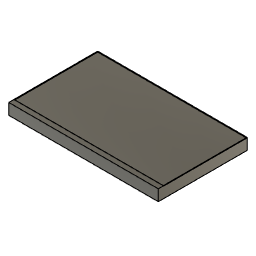
Final product (Autodesk Fusion 360 archive; units mm, degrees)
design "Écran 1"
Autodesk Fusion 360 part; units mm, degrees
sketch "Esquisse1" plane through (0, 0, 0) normal (0, 0, 1) x (1, 0, 0)
  line L0 (269, 160) -> (-269, 160)
  line L1 (-269, 160) -> (-269, -160)
  line L2 (-269, -160) -> (269, -160)
  line L3 (269, -160) -> (269, 160)
  line L4 (269, 160) -> (-269, -160) construction
  line L5 (-269, 160) -> (269, -160) construction
  dimension "d1" = 538
  dimension "d2" = 320
  constraint horizontal L0
  constraint perpendicular L0 L1
  constraint parallel L0 L2
  constraint parallel L1 L3
  constraint coincident L4 origin
  constraint coincident L5 origin
  measures "d1" distance of L1.end L2.end
  measures "d2" distance of L0.end L1.end
extrude "Extrusion1" add sketch "Esquisse1" along normal blind 40 makes body 1
sketch "Esquisse2" plane through (0, 0, 40) normal (0, 0, 1) x (-1, 0, 0)
  line L0 (-269, 160) -> (-269, -160)
  line L1 (-269, -160) -> (269, -160)
  line L2 (269, -160) -> (269, 160)
  line L3 (269, 160) -> (-269, 160)
  line L4 (268, -159) -> (-268, -159)
  line L5 (-268, -159) -> (-268, 141)
  line L6 (-268, 141) -> (268, 141)
  line L7 (268, 141) -> (268, -159)
  dimension "d5" = 536
  dimension "d6" = 300
  dimension "d7" = 1
  dimension "d8" = 1
  constraint horizontal L4
  constraint vertical L5
  constraint horizontal L6
  constraint vertical L7
  measures "d5" distance of L4.start L4.end
  measures "d6" distance of L4.start L6.end
  measures "d7" distance of L1 L4
  measures "d8" distance of L2 L7
extrude "Extrusion2" cut sketch "Esquisse2" against normal blind 2 contours L4 L5 L6 L7 bodies 1
sketch "Esquisse3" plane through (0, 0, 0) normal (0, 0, -1) x (1, 0, 0)
  line L0 (269, -160) -> (269, 160)
  line L1 (269, 160) -> (-269, 160)
  line L2 (-269, 160) -> (-269, -160)
  line L3 (-269, -160) -> (269, -160)
  circle A0 centre (-49, 20) radius 1.25
  circle A1 centre (51, 20) radius 1.25
  circle A2 centre (-49, -80) radius 1.25
  circle A3 centre (51, -80) radius 1.25
  dimension "d11" = 2.5
  dimension "d12" = 2.5
  dimension "d13" = 2.5
  dimension "d14" = 2.5
  dimension "d15" = 140
  dimension "d16" = 140
  dimension "d17" = 100
  dimension "d18" = 100
  dimension "d19" = 100
  dimension "d20" = 100
  dimension "d21" = 220
  dimension "d22" = 220
  measures "d11" diameter of A0
  measures "d12" diameter of A1
  measures "d13" diameter of A2
  measures "d14" diameter of A3
  measures "d15" distance of L1 A0.centre
  measures "d16" distance of L1 A1.centre
  measures "d17" distance of A0.centre A1.centre
  measures "d18" vertical distance of A0.centre A2.centre
  measures "d19" horizontal distance of A2.centre A3.centre
  measures "d20" vertical distance of A1.centre A3.centre
  measures "d21" distance of L2 A0.centre
  measures "d22" distance of L2 A2.centre
hole "Perçage1" at (-49, -20, 0) at (51, -20, 0) at (51, 80, 0) at (-49, 80, 0) direction (0, 0, 1) diameter 2.5 depth 20 tip angle 180 bodies 1
thread "Filetage1" "ISO Metric profile 2.5 M2.5x0.45 6H" major diameter 2.58 minor diameter 2.0755 pitch 0.45 angle 60 resizes the face on face at (-48.5725, -21.1746, 6.6667) on bodies 1
thread "Filetage2" "ISO Metric profile 2.5 M2.5x0.45 6H" major diameter 2.58 minor diameter 2.0755 pitch 0.45 angle 60 resizes the face on face at (51.4275, -21.1746, 6.6667) on bodies 1
thread "Filetage3" "ISO Metric profile 2.5 M2.5x0.45 6H" major diameter 2.58 minor diameter 2.0755 pitch 0.45 angle 60 resizes the face on face at (49.8151, 80.3981, 13.3333) on bodies 1
thread "Filetage4" "ISO Metric profile 2.5 M2.5x0.45 6H" major diameter 2.58 minor diameter 2.0755 pitch 0.45 angle 60 resizes the face on face at (-50.1849, 80.3981, 13.3333) on bodies 1
sketch "Esquisse4" plane through (0, 0, 0) normal (0, 0, -1) x (1, 0, 0)
  circle A0 centre (51, -80) radius 1.0377
  circle A1 centre (-49, 20) radius 1.0377
  circle A2 centre (51, 20) radius 1.0377
  circle A3 centre (-49, -80) radius 1.0377
  line L0 (269, -160) -> (269, 160)
  line L1 (269, 160) -> (-269, 160)
  line L2 (-269, 160) -> (-269, -160)
  line L3 (-269, -160) -> (269, -160)
  line L4 (-37, -112) -> (13, -112)
  line L5 (13, -112) -> (13, -102)
  line L6 (13, -102) -> (-37, -102)
  line L7 (-37, -102) -> (-37, -112)
  line L8 (63, -102) -> (73, -102)
  line L9 (73, -102) -> (73, -112)
  line L10 (73, -112) -> (63, -112)
  line L11 (63, -112) -> (63, -102)
  circle A4 centre (68, -107) radius 2.5
  circle A5 centre (-34.4, -107) radius 2.5
  circle A6 centre (10.4, -107) radius 2.5
  dimension "d26" = 50
  dimension "d27" = 10
  dimension "d28" = 22
  dimension "d29" = 12
  dimension "d30" = 10
  dimension "d31" = 10
  dimension "d32" = 22
  dimension "d33" = 12
  dimension "d34" = 5
  dimension "d35" = 5
  dimension "d36" = 5
  dimension "d37" = 5
  dimension "d38" = 5
  dimension "d39" = 5
  dimension "d40" = 5
  dimension "d42" = 2.6
  dimension "d43" = 2.6
  constraint horizontal L4
  constraint vertical L5
  constraint horizontal L6
  constraint vertical L7
  constraint horizontal L8
  constraint vertical L9
  constraint horizontal L10
  constraint vertical L11
  measures "d26" distance of L4.start L4.end
  measures "d27" distance of L4.start L6.end
  measures "d28" distance of A3.centre L6
  measures "d29" distance of A3.centre L7
  measures "d30" distance of L8.start L8.end
  measures "d31" distance of L8.start L10.end
  measures "d32" distance of A0.centre L8
  measures "d33" distance of A0.centre L11
  measures "d34" diameter of A4
  measures "d35" distance of L8 A4.centre
  measures "d36" distance of L11 A4.centre
  measures "d37" diameter of A5
  measures "d38" diameter of A6
  measures "d39" distance of L6 A5.centre
  measures "d40" distance of L6 A6.centre
  measures "d42" distance of L7 A5.centre
  measures "d43" distance of L5 A6.centre
extrude "Extrusion3" add sketch "Esquisse4" along normal blind 10 separate body contours L4 L5 L6 L7 | L8 L9 L10 L11 makes body 2 at (-3.6667, 102, -3.3333) makes body 3 at (65.6508, 107.8551, -6.6667)
sketch "Esquisse5" plane through (0, 112, 0) normal (0, 1, 0) x (-1, 0, 0)
  line L0 (37, 0) -> (-13, 0)
  line L1 (-13, 0) -> (-13, -10)
  line L2 (-13, -10) -> (37, -10)
  line L3 (37, -10) -> (37, 0)
  line L4 (17, -2.5) -> (27, -2.5)
  line L5 (27, -2.5) -> (27, -7.5)
  line L6 (27, -7.5) -> (17, -7.5)
  line L7 (17, -7.5) -> (17, -2.5)
  dimension "d46" = 10
  dimension "d47" = 5
  dimension "d48" = 10
  dimension "d49" = 2.5
  constraint horizontal L4
  constraint vertical L5
  constraint horizontal L6
  constraint vertical L7
  measures "d46" distance of L4.start L4.end
  measures "d47" distance of L4.start L6.end
  measures "d48" distance of L3 L5
  measures "d49" distance of L2 L6
extrude "Extrusion4" cut sketch "Esquisse5" against normal blind 5 contours L4 L5 L6 L7 bodies 2

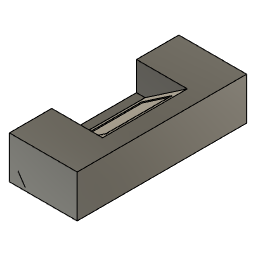
design "Socle partie inférieur"
Autodesk Fusion 360 part; units mm, degrees
sketch "Esquisse1" plane through (0, 0, 0) normal (0, 1, 0) x (1, 0, 0)
  line L0 (0, 0) -> (120, 0)
  line L1 (120, 0) -> (120, -100)
  line L2 (120, -100) -> (0, -100)
  line L3 (0, -100) -> (0, 0)
  line L4 (0, 0) -> (37.2, 0)
  line L5 (37.2, 0) -> (37.2, -32.2)
  line L6 (37.2, -32.2) -> (0, -32.2)
  line L7 (0, -32.2) -> (0, 0)
  line L8 (37.2, -32.2) -> (20.4, -32.2)
  line L9 (37.2, -7.4) -> (37.2, -32.2)
  line L10 (20.4, -32.2) -> (37.2, -7.4)
  line L11 (120, -100) -> (20.4, -32.2)
  line L12 (20.4, -32.2) -> (37.256, -7.4381)
  line L13 (37.256, -7.4381) -> (136.856, -75.2381)
  line L14 (136.856, -75.2381) -> (120, -100)
  line L15 (120, -100) -> (120, 0)
  line L16 (120, 0) -> (160, 0)
  line L17 (160, 0) -> (160, -100)
  line L18 (160, -100) -> (120, -100)
  line L19 (37.2, -7.4) -> (37.2, 0)
  line L20 (37.2, 0) -> (160, 0)
  line L21 (160, 0) -> (160, -7.4)
  line L22 (160, -7.4) -> (37.2, -7.4)
  line L23 (160, -7.4) -> (160, -100)
  line L24 (160, -100) -> (120, -100)
  line L25 (120, -100) -> (120, -7.4)
  line L26 (120, -7.4) -> (160, -7.4)
  dimension "d1" = 120
  dimension "d2" = 100
  dimension "d3" = 37.2
  dimension "d4" = 32.2
  dimension "d11" = 16.8
  dimension "d12" = 24.8
  dimension "d19" = 40
  constraint horizontal L0
  constraint vertical L1
  constraint horizontal L2
  constraint vertical L3
  constraint coincident L0.start L3.end
  constraint horizontal L4
  constraint vertical L5
  constraint horizontal L6
  constraint vertical L7
  constraint horizontal L8
  constraint vertical L9
  constraint perpendicular L11 L12
  constraint parallel L11 L13
  constraint parallel L12 L14
  constraint perpendicular L15 L16
  constraint parallel L15 L17
  constraint parallel L16 L18
  constraint perpendicular L19 L20
  constraint parallel L19 L21
  constraint parallel L20 L22
  constraint perpendicular L23 L24
  constraint parallel L23 L25
  constraint parallel L24 L26
  constraint perpendicular L22 L23
  measures "d1" distance of L0.start L0.end
  measures "d2" distance of L0.start L2.end
  measures "d3" distance of L0.start L4.end
  measures "d4" distance of L0.start L6.end
  measures "d11" distance of L5.end L8.end
  measures "d12" distance of L5.end L9.start
  measures "d19" distance of L1.end L17.end
extrude "Extrusion3" add sketch "Esquisse1" along normal blind 200 contours L0 L3 L4 L5 L6 L7 L10 L19 | L0 L1 L5 L15 L19 L20 L22 | L1 L15 L16 L17 L20 L21 L22 L26 | L5 L6 L8 L9 L12 | L1 L5 L6 L8 L9 L11 L12 L13 L15 L25 | L1 L13 L14 L15 L17 L18 L22 L23 L24 L25 L26 | L1 L13 L14 L15 L25
extrude "Extrusion4" add sketch "Esquisse1" along normal blind 100 contours L0 L1 L5 L15 L19 L20 L22 | L2 L3 L6 L11 | L1 L15 L16 L17 L20 L21 L22 L26 | L1 L5 L9 L12 L13 L15 L22 L25 | L1 L13 L14 L15 L17 L18 L22 L23 L24 L25 L26
mirror "Symétrie miroir2" about plane through (0, 200, 0) normal (0, 1, 0) of bodies 1 merged
sketch "Esquisse3" plane through (-8.5188, 0, 12.5143) normal (-0.562719, 0, 0.826649) x (0, -1, 0)
  line L0 (-100, 34.9832) -> (-100, 155.4697)
  line L1 (-100, 155.4697) -> (-300, 155.4697)
  line L2 (-300, 155.4697) -> (-300, 34.9832)
  line L3 (-300, 34.9832) -> (-100, 34.9832)
  line L4 (-277.5, 138.4697) -> (-122.5, 138.4697)
  line L5 (-122.5, 138.4697) -> (-122.5, 52.4697)
  line L6 (-122.5, 52.4697) -> (-277.5, 52.4697)
  line L7 (-277.5, 52.4697) -> (-277.5, 138.4697)
  line L8 (-277.5, 138.4697) -> (-122.5, 52.4697) construction
  line L9 (-122.5, 138.4697) -> (-277.5, 52.4697) construction
  point P0 (-200, 95.4697)
  dimension "d22" = 155
  dimension "d23" = 86
  dimension "d24" = 22.5
  dimension "d25" = 17
  constraint horizontal L4
  constraint perpendicular L4 L5
  constraint parallel L4 L6
  constraint parallel L5 L7
  constraint coincident L8 P0
  constraint coincident L9 P0
  measures "d22" distance of L5.end L6.end
  measures "d23" distance of L4.end L5.end
  measures "d24" distance of L2 L7
  measures "d25" distance of L1 L4
extrude "Extrusion6" cut sketch "Esquisse3" against normal blind 2 contours L4 L5 L6 L7
